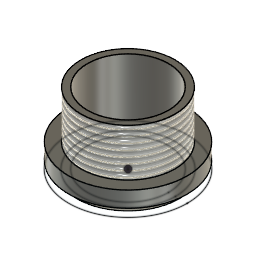
Microphone_sensor_water_leader (Autodesk Fusion 360 design; units mm, degrees)
part number: 2026-04-09-10-56-57-703
Autodesk Fusion 360 part; units mm, degrees
sketch "Sketch1" plane through (0, 0, 0) normal (0, 0, 1) x (1, 0, 0)
  circle A0 centre (0, 0) radius 5.125
  circle A1 centre (0, 0) radius 6
  circle A2 centre (0, 0) radius 7.5
  dimension "d1" = 10.25
  dimension "d2" = 12
  dimension "d3" = 15
  constraint coincident A0.centre A1.centre
  constraint concentric A0 A1
  constraint concentric A0 A2
  measures "d1" diameter of A0
  measures "d2" diameter of A1
  measures "d3" diameter of A2
extrude "Extrude1" add sketch "Sketch1" along normal blind 3 contours A2
extrude "Extrude2" add sketch "Sketch1" along normal blind 9 contours A1
chamfer "Chamfer1" distance 1 angle 45 1 edges at (-6.9925, -2.7121, 0)
thread "Thread1" "ISO Metric profile 12.0 M12x0.75 M12x0.75 6g" major diameter 11.908 minor diameter 11.0445 pitch 0.75 angle 60 resizes the face on face at (5.9702, -0.5974, 5)
